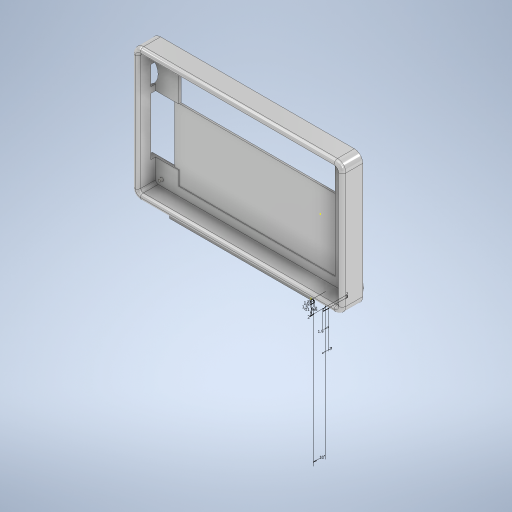
# Autodesk Inventor part: monitor-stand
Saved by Autodesk Inventor 2023 (Build 270158030, 158C)
## iProperties
Created: 2024-02-27
Part Number: monitor-stand
Material: Generic
Document SubType Name: Modeling
Designer: Imogen Heard
Density: 1 g/cm^3
Appearance: Expanded Metal 01
Author: Imogen Heard
Autodesk Inventor part; units mm, degrees
ref_plane "YZ Plane" through (0, 0, 0) normal (1, 0, 0) x (0, 1, 0)
ref_plane "XZ Plane" through (0, 0, 0) normal (0, 1, 0) x (-1, 0, 0)
ref_plane "XY Plane" through (0, 0, 0) normal (0, 0, 1) x (1, 0, 0)
sketch "Sketch1" plane through (0, 0, 0) normal (0, 0, 1) x (1, 0, 0)
  line L0 (-82.5, 50) -> (82.5, 50)
  line L1 (82.5, 50) -> (82.5, -50)
  line L2 (82.5, -50) -> (-82.5, -50)
  line L3 (-82.5, -50) -> (-82.5, 50)
  point P0 (0, 0)
  dimension "d0" = 165
  dimension "d1" = 100
  dimension "d2" = 82.5
  dimension "d3" = 50
  constraints: 8 end point, 2 parallel, 1 horizontal, 1 perpendicular
  measures "d0" distance between parallel lines of L1 L3
  measures "d1" distance between parallel lines of L2 L0
  measures "d2" horizontal distance of L2.end point (0, 0)
  measures "d3" distance from line of L2 point (0, 0)
extrude "Extrusion1" add sketch "Sketch1" along normal blind 8.36
sketch "Sketch2" plane through (0, 0, 0) normal (0, 0, -1) x (-1, 0, 0)
  circle A0 centre (-77.5, 45) radius 2.75
  circle A1 centre (77.5, 45) radius 2.75
  circle A2 centre (77.5, -45) radius 2.75
  circle A3 centre (-77.5, -45) radius 2.75
  line L0 (-82.5, 50) -> (82.5, 50) projected
  line L1 (-82.5, -50) -> (-82.5, 50) projected
  line L2 (82.5, -50) -> (-82.5, -50) projected
  line L3 (82.5, 50) -> (82.5, -50) projected
  point P0 (0, 0)
  dimension "d6" = 5.5
  dimension "d7" = 5
  dimension "d8" = 5
  dimension "d9" = 5
  dimension "d10" = 5
  constraints: 4 centre point, 3 equal radius, 2 horizontal alignment, 2 vertical alignment
  measures "d6" diameter of A3
  measures "d7" distance from line of L0 A0.centre
  measures "d8" distance from line of L1 A0.centre
  measures "d9" distance from line of L2 A3.centre
  measures "d10" distance from line of L3 A2.centre
extrude "Extrusion2" add sketch "Sketch2" along normal blind 4 contours A0 | A1 | A2 | A3
hole "Hole1" at (-77.5, -45, -4) direction (0, 0, 1) diameter 2.013 depth 4 tip angle 118 start extended yes countersink diameter 4 countersink angle 90 thread size "M2.5x0.45" class "6H" standard "ISO Metric profile"
hole "Hole2" at (77.5, 45, -4) direction (0, 0, 1) diameter 2.013 depth 4 tip angle 118 start extended yes countersink diameter 4 countersink angle 90 thread size "M2.5x0.45" class "6H" standard "ISO Metric profile"
hole "Hole3" at (77.5, -45, -4) direction (0, 0, 1) diameter 2.013 depth 4 tip angle 118 start extended yes countersink diameter 4 countersink angle 90 thread size "M2.5x0.45" class "6H" standard "ISO Metric profile"
hole "Hole4" at (-77.5, 45, -4) direction (0, 0, 1) diameter 2.013 depth 4 tip angle 118 start extended yes countersink diameter 4 countersink angle 90 thread size "M2.5x0.45" class "6H" standard "ISO Metric profile"
fillet "Fillet1" radius 2 4 edges at (82.5, 50, 4.18) (-82.5, 50, 4.18) (82.5, -50, 4.18) (-82.5, -50, 4.18)
sketch "Sketch4" plane through (0, 0, 0) normal (0, 0, -1) x (-1, 0, 0)
  line L0 (81.5, 35) -> (73.35, 35)
  line L1 (73.35, 35) -> (73.35, 23)
  line L2 (73.35, 23) -> (81.5, 23)
  line L3 (81.5, 23) -> (81.5, 35)
  line L4 (-80.5, 50) -> (80.5, 50) projected
  line L5 (82.5, 48) -> (82.5, -48) projected
  point P0 (0, 0)
  dimension "d54" = 15
  dimension "d55" = 12
  dimension "d56" = 9.15
  dimension "d57" = 1
  constraints: 8 end point, 2 parallel, 1 horizontal, 1 perpendicular
  measures "d54" distance between parallel lines of L0 L4
  measures "d55" distance between parallel lines of L2 L0
  measures "d56" distance between parallel lines of L5 L1
  measures "d57" distance between parallel lines of L5 L3
extrude "Extrusion3" add sketch "Sketch4" along normal blind 3
fillet "Fillet2" radius 6 2 edges at (-81.5, 35, -1.5) (-81.5, 23, -1.5)
sketch "Sketch5" plane through (0, 0, 0) normal (0, 0, -1) x (-1, 0, 0)
  arc A0 (77.425, 21.5) -> (77.425, 36.5) centre (77.425, 29) ccw
  line L0 (73.35, 35) -> (73.35, 23) projected
  line L1 (73.35, 23) -> (75.5, 23) projected
  line L2 (75.5, 35) -> (73.35, 35) projected
  line L3 (81.5, 35) -> (73.35, 35) projected
  line L4 (77.425, 36.5) -> (77.425, 21.5)
  arc A1 (75.5, 23) -> (75.5, 35) centre (75.5, 29) ccw projected
  point P0 (0, 0)
  point P1 (77.425, 35)
  point P2 (77.425, 35)
  point P3 (77.425, 23)
  point P4 (77.425, 34.6828)
  point P5 (77.425, 23.3172)
  point P6 (77.425, 35)
  dimension "d60" = 15
  dimension "d61" = 12
  dimension "d62" = 6
  dimension "d64" = 4.075
  constraints: 2 end point, 2 point on circle, 1 centre point, 1 midpoint
  measures "d60" diameter of A0
  measures "d61" distance from line of point (77.425, 35) L1
  measures "d62" distance from line of L1 A0.centre
  measures "d64" distance from line of L0 A0.centre
extrude "Extrusion4" add sketch "Sketch5" along normal blind 2.7 contours L4 A1 A0 | L4 A1
sketch "Sketch6" plane through (-82.5, -48, 8.36) normal (-1, 0, 0) x (0, 0, 1)
  line L0 (-14.66, 18.5) -> (-10.47, 18.5)
  line L1 (-10.47, 33.5) -> (-14.66, 33.5)
  line L2 (-14.66, 33.5) -> (-14.66, 18.5)
  line L3 (-10.47, 20) -> (-9.06, 21)
  line L4 (-9.06, 21) -> (-9.06, 31)
  line L5 (-8.36, 0) -> (-8.36, 96) projected
  line L6 (-9.06, 31) -> (-10.47, 32)
  line L7 (-10.47, 33) -> (-8.36, 33)
  line L8 (-8.36, 33) -> (-8.36, 33.5)
  line L9 (-8.36, 33.5) -> (-10.47, 33.5)
  line L10 (-10.47, 18.5) -> (-8.36, 18.5)
  line L11 (-8.36, 18.5) -> (-8.36, 19)
  line L12 (-8.36, 19) -> (-10.47, 19)
  line L13 (-8.36, -2) -> (0, -2) projected
  line L14 (-10.47, 19) -> (-10.47, 20)
  line L15 (-10.47, 32) -> (-10.47, 33)
  line L16 (-10.92, 33.05) -> (-10.92, 31.7675)
  line L17 (-10.92, 31.7675) -> (-9.51, 30.7675)
  line L18 (-9.51, 30.7675) -> (-9.51, 21.2325)
  line L19 (-9.51, 21.2325) -> (-10.92, 20.2325)
  line L20 (-10.92, 20.2325) -> (-10.92, 18.95)
  line L21 (-10.92, 18.95) -> (-14.21, 18.95)
  line L22 (-14.21, 18.95) -> (-14.21, 33.05)
  line L23 (-14.21, 33.05) -> (-10.92, 33.05)
  point P0 (-8.36, 48)
  point P1 (-12.565, 33.05)
  point P2 (-10.47, 32.5)
  point P3 (-10.47, 19.5)
  point P4 (-8.36, 18.5)
  point P5 (-10.47, 33.5)
  dimension "d68" = 0.5
  dimension "d69" = 0.5
  dimension "d70" = 15
  dimension "d71" = 6.3
  dimension "d73" = 0.7
  dimension "d74" = 1.5
  dimension "d75" = 1.5
  dimension "d76" = 20.5
  dimension "d77" = 2.5
  dimension "d78" = 2.5
  dimension "d79" = 2.11
  dimension "d80" = 0.45
  dimension "d81" = 0.45
  dimension "d82" = 0.45
  dimension "d83" = 0.45
  dimension "d84" = 0.45
  dimension "d85" = 0.45
  constraints: 44 end point, 9 parallel, 6 perpendicular, 3 horizontal, 3 midpoint, 2 point on line, 1 coincident, 1 vertical alignment, 2 other
  measures "d68" distance between parallel lines of L9 L7
  measures "d69" distance between parallel lines of L12 L10
  measures "d70" distance between parallel lines of L1 L0
  measures "d71" distance between parallel lines of L5 L2
  measures "d73" distance between parallel lines of L5 L4
  measures "d74" distance from line of L1 L6.end
  measures "d75" distance from line of L0 L3.start
  measures "d76" distance between parallel lines of L13 L0
  measures "d77" distance from line of L1 L4.end
  measures "d78" distance from line of L0 L3.end
  measures "d79" distance between parallel lines of L5 L15
  measures "d80" distance between parallel lines of L2 L22
  measures "d81" distance from line of L1 point (-12.565, 33.05)
  measures "d82" distance between parallel lines of L4 L18
  measures "d83" distance from line of point (-10.47, 32.5) L16
  measures "d84" distance between parallel lines of L0 L21
  measures "d85" distance from line of point (-10.47, 19.5) L20
extrude "Extrusion5" add sketch "Sketch6" along normal blind 0.4 and the other way blind 12 contours L2 L1 L9 L5 L7 L15 L6 L4 L3 L14 L12 L10 L0
fillet "Fillet3" radius 0.5 6 edges at (-76.7, -14.5, -6.3) (-76.7, -29.5, -6.3) (-76.7, -27.7675, -2.56) (-76.7, -16.2325, -2.56) (-76.7, -17, -0.7) (-76.7, -27, -0.7)
fillet "Fillet4" radius 0.2 8 edges at (-76.7, -29.05, -5.85) (-76.7, -14.95, -5.85) (-76.7, -29.05, -2.56) (-76.7, -26.7675, -1.15) (-76.7, -17.2325, -1.15) (-76.7, -14.95, -2.56) (-76.7, -16, -2.11) (-76.7, -28, -2.11)
sketch "Sketch7" plane through (-70.5, -48, 8.36) normal (-1, 0, 0) x (0, 0, -1)
  arc A0 (9.2708, -20.8505) -> (9.06, -21.2584) centre (9.56, -21.2584) ccw projected
  line L0 (10.3857, -20.0598) -> (9.2708, -20.8505) projected
  arc A1 (10.3857, -20.0598) -> (10.47, -19.8967) centre (10.27, -19.8967) ccw projected
  line L1 (10.47, -19) -> (10.47, -19.8967) projected
  line L2 (8.36, -19) -> (10.47, -19) projected
  line L3 (14.16, -18.5) -> (8.36, -18.5) projected
  arc A2 (14.66, -19) -> (14.16, -18.5) centre (14.16, -19) ccw projected
  line L4 (14.66, -33) -> (14.66, -19) projected
  arc A3 (14.16, -33.5) -> (14.66, -33) centre (14.16, -33) ccw projected
  line L5 (8.36, -33.5) -> (14.16, -33.5) projected
  line L6 (10.47, -33) -> (8.36, -33) projected
  line L7 (10.47, -32.1033) -> (10.47, -33) projected
  arc A4 (10.47, -32.1033) -> (10.3857, -31.9402) centre (10.27, -32.1033) ccw projected
  line L8 (9.2708, -31.1495) -> (10.3857, -31.9402) projected
  arc A5 (9.06, -30.7416) -> (9.2708, -31.1495) centre (9.56, -30.7416) ccw projected
  line L9 (9.06, -21.2584) -> (9.06, -30.7416) projected
  arc A6 (10.92, -32.0258) -> (10.7092, -31.618) centre (10.42, -32.0258) ccw projected
  line L10 (10.92, -32.85) -> (10.92, -32.0258) projected
  arc A7 (10.92, -32.85) -> (11.12, -33.05) centre (11.12, -32.85) ccw projected
  line L11 (14.01, -33.05) -> (11.12, -33.05) projected
  arc A8 (14.01, -33.05) -> (14.21, -32.85) centre (14.01, -32.85) ccw projected
  line L12 (14.21, -19.15) -> (14.21, -32.85) projected
  arc A9 (14.21, -19.15) -> (14.01, -18.95) centre (14.01, -19.15) ccw projected
  line L13 (11.12, -18.95) -> (14.01, -18.95) projected
  arc A10 (11.12, -18.95) -> (10.92, -19.15) centre (11.12, -19.15) ccw projected
  line L14 (10.92, -19.9742) -> (10.92, -19.15) projected
  arc A11 (10.7092, -20.382) -> (10.92, -19.9742) centre (10.42, -19.9742) ccw projected
  line L15 (9.5943, -21.1727) -> (10.7092, -20.382) projected
  arc A12 (9.5943, -21.1727) -> (9.51, -21.3359) centre (9.71, -21.3359) ccw projected
  line L16 (9.51, -30.6641) -> (9.51, -21.3359) projected
  arc A13 (9.51, -30.6641) -> (9.5943, -30.8273) centre (9.71, -30.6641) ccw projected
  line L17 (10.7092, -31.618) -> (9.5943, -30.8273) projected
  line L18 (8.36, -33) -> (8.36, -33.5) projected
  line L19 (8.36, -18.5) -> (8.36, -19) projected
  point P0 (8.36, -48)
extrude "Extrusion6" add sketch "Sketch7" along normal blind 4.5 contours A6 L17 A13 L16 A12 L15 A11 L14 A10 L13 A9 L12 A8 L11 A7 L10
sketch "Sketch8" plane through (-82.5, -48, 8.36) normal (-1, 0, 0) x (0, 0, 1)
  line L0 (-10.06, 42.6) -> (-10.06, 48.5) construction
  line L1 (-8.46, 42.6) -> (-8.46, 48.5)
  line L2 (-11.66, 48.5) -> (-11.66, 42.6)
  arc A0 (-11.66, 42.6) -> (-8.46, 42.6) centre (-10.06, 42.6) ccw
  arc A1 (-8.46, 48.5) -> (-11.66, 48.5) centre (-10.06, 48.5) ccw
  line L3 (-8.36, 71.4778) -> (-8.36, 33.5) projected
  line L4 (-11.31, 42.6) -> (-11.31, 48.5)
  arc A2 (-8.81, 48.5) -> (-11.31, 48.5) centre (-10.06, 48.5) ccw
  line L5 (-8.81, 48.5) -> (-8.81, 42.6)
  arc A3 (-11.31, 42.6) -> (-8.81, 42.6) centre (-10.06, 42.6) ccw
  point P0 (-8.36, 48)
  point P1 (-10.06, 45.55)
  point P2 (-10.06, 50.1)
  point P3 (-10.06, 41)
  point P4 (-8.36, -2)
  dimension "d94" = 9.1
  dimension "d95" = 3.2
  dimension "d96" = 0.1
  dimension "d97" = 43
  dimension "d98" = 0.35
  constraints: 12 end point, 10 point on circle, 4 centre point, 4 tangent, 2 parallel, 1 midpoint, 1 vertical, 3 other
  measures "d94" distance of point (-10.06, 50.1) point (-10.06, 41)
  measures "d95" distance between parallel lines of L1 L2
  measures "d96" distance between parallel lines of L3 L1
  measures "d97" vertical distance of point (-8.36, -2) point (-10.06, 41)
  measures "d98" distance between parallel lines of L2 L4
extrude "Extrusion7" add sketch "Sketch8" against normal blind 7.5
sketch "Sketch9" plane through (-75, -48, 8.36) normal (1, 0, 0) x (0, 0, -1)
  arc A0 (11.66, 48.5) -> (8.46, 48.5) centre (10.06, 48.5) ccw projected
  line L0 (8.46, 48.5) -> (8.46, 42.6) projected
  arc A1 (8.46, 42.6) -> (11.66, 42.6) centre (10.06, 42.6) ccw projected
  line L1 (11.66, 42.6) -> (11.66, 48.5) projected
  line L2 (8.81, 42.6) -> (8.81, 48.5) projected
  arc A2 (11.31, 48.5) -> (8.81, 48.5) centre (10.06, 48.5) ccw projected
  line L3 (11.31, 48.5) -> (11.31, 42.6) projected
  arc A3 (8.81, 42.6) -> (11.31, 42.6) centre (10.06, 42.6) ccw projected
  point P0 (8.36, 48)
extrude "Extrusion8" add sketch "Sketch9" against normal blind 2 contours L2 A2 L3 A3
sketch "Sketch10" plane through (-82.5, -48, 8.36) normal (-1, 0, 0) x (0, 0, 1)
  circle A0 centre (-10.91, 59) radius 2.45
  circle A1 centre (-10.91, 59) radius 1.72
  line L0 (-8.36, 71.4778) -> (-8.36, 33.5) projected
  line L1 (0, 98) -> (-8.36, 98) projected
  point P0 (-8.36, 48)
  dimension "d103" = 4.9
  dimension "d104" = 0.73
  dimension "d105" = 2.55
  dimension "d106" = 39
  constraints: 2 centre point, 1 concentric
  measures "d103" diameter of A0
  measures "d104" radial gap between concentric circles of A0 A1
  measures "d105" distance from line of L0 A0.centre
  measures "d106" distance from line of L1 A0.centre
extrude "Extrusion9" add sketch "Sketch10" against normal blind 14
sketch "Sketch11" plane through (-68.5, 11, -2.55) normal (1, 0, 0) x (0, 0, -1)
  line L0 (-2.55, 12.4778) -> (-2.55, -25.5) projected
  line L1 (2.45, 3.175) -> (-2.55, 3.175)
  line L2 (-2.55, 3.175) -> (-2.55, -3.175)
  line L3 (-2.55, -3.175) -> (2.45, -3.175)
  line L4 (2.45, -3.175) -> (2.45, 3.175)
  circle A0 centre (0, 0) radius 1.72 projected
  point P0 (-2.55, -11)
  point P1 (-2.55, 3.175)
  dimension "d109" = 6.35
  dimension "d110" = 3.175
  dimension "d111" = 5
  constraints: 8 end point, 2 parallel, 1 horizontal, 1 perpendicular, 1 point on line
  measures "d109" distance between parallel lines of L3 L1
  measures "d110" distance from line of A0.centre L3
  measures "d111" distance between parallel lines of L0 L4
extrude "Extrusion10" add sketch "Sketch11" against normal blind 12
sketch "Sketch12" plane through (0, 0, 0) normal (0, 0, -1) x (-1, 0, 0)
  line L0 (-63.9, 42.33) -> (-25.9, 42.33)
  line L1 (-25.9, 42.33) -> (-25.9, 24.33)
  line L2 (-25.9, 24.33) -> (-63.9, 24.33)
  line L3 (-63.9, 24.33) -> (-63.9, 42.33)
  line L4 (22.83, 42.33) -> (60.83, 42.33)
  line L5 (60.83, 42.33) -> (60.83, 24.33)
  line L6 (60.83, 24.33) -> (22.83, 24.33)
  line L7 (22.83, 24.33) -> (22.83, 42.33)
  line L8 (-82.5, -48) -> (-82.5, 48) projected
  line L9 (-80.5, 50) -> (80.5, 50) projected
  line L10 (82.5, 48) -> (82.5, 34.5222) projected
  point P0 (0, 0)
  dimension "d114" = 38
  dimension "d115" = 18
  dimension "d116" = 38
  dimension "d117" = 18.6
  dimension "d118" = 7.67
  dimension "d119" = 21.67
  constraints: 16 end point, 4 parallel, 2 horizontal, 2 horizontal alignment, 2 perpendicular, 2 point on line
  measures "d114" distance between parallel lines of L1 L3
  measures "d115" distance between parallel lines of L2 L0
  measures "d116" distance between parallel lines of L5 L7
  measures "d117" distance between parallel lines of L8 L3
  measures "d118" distance between parallel lines of L9 L0
  measures "d119" distance between parallel lines of L5 L10
extrude "Extrusion11" add sketch "Sketch12" along normal blind 5.09
fillet "Fillet5" radius 3 8 edges at (63.9, 24.33, -2.545) (63.9, 42.33, -2.545) (25.9, 24.33, -2.545) (25.9, 42.33, -2.545) (-60.83, 42.33, -2.545) (-22.83, 42.33, -2.545) (-22.83, 24.33, -2.545) (-60.83, 24.33, -2.545)
fillet "Fillet6" radius 0.2 16 edges at (-23.7087, 41.4513, -5.09) (-22.83, 33.33, -5.09) (-23.7087, 25.2087, -5.09) (-41.83, 24.33, -5.09) (-59.9513, 25.2087, -5.09) (-60.83, 33.33, -5.09) (-59.9513, 41.4513, -5.09) (-41.83, 42.33, -5.09) (26.7787, 41.4513, -5.09) (44.9, 42.33, -5.09) (63.0213, 41.4513, -5.09) (63.9, 33.33, -5.09) (63.0213, 25.2087, -5.09) (44.9, 24.33, -5.09) (26.7787, 25.2087, -5.09) (25.9, 33.33, -5.09)
sketch "Sketch13" plane through (77.5, 45, -4) normal (0, 0, -1) x (-1, 0, 0)
  line L0 (-10, 10) -> (165, 10)
  line L1 (165, 10) -> (165, -100)
  line L2 (165, -100) -> (-10, -100)
  line L3 (-10, -100) -> (-10, 10)
  line L4 (-3, 5) -> (158, 5) projected
  line L5 (-5, -93) -> (-5, 3) projected
  line L6 (160, -21.5222) -> (160, -59.5) projected
  line L7 (158, -95) -> (-3, -95) projected
  line L8 (11, -2) -> (141, -2)
  line L9 (141, -88) -> (11, -88)
  line L10 (141, -88) -> (141, -2)
  line L11 (141, -29.8869) -> (141, -2)
  line L12 (160, 3) -> (160, -93) projected
  line L13 (160, -39.175) -> (160, -57.5)
  line L14 (160, -74.5) -> (160, -93) projected
  line L15 (11, -2) -> (11, -88)
  line L16 (146, -37.175) -> (146, -30.825) projected
  line L17 (144, -28.825) -> (144, -39.175)
  line L18 (146, -57.5) -> (146, -76.5)
  line L19 (146, -30.825) -> (158, -30.825) projected
  line L20 (146, -37.175) -> (158, -37.175) projected
  line L21 (160.4, -59.5) -> (148, -59.5) projected
  line L22 (148, -74) -> (148, -60) projected
  line L23 (160, -74.5) -> (148, -74.5) projected
  line L24 (144, -28.825) -> (165, -28.825)
  line L25 (144, -39.175) -> (165, -39.175)
  line L26 (146, -76.5) -> (165, -76.5)
  line L27 (146, -57.5) -> (165, -57.5)
  arc A0 (165, -6) -> (165, -26) centre (169.6, -16) ccw
  line L28 (150.85, -10) -> (150.85, -22) projected
  line L29 (141, -28.825) -> (160, -28.825)
  line L30 (160, -28.825) -> (160, -76.5)
  line L31 (160, -76.5) -> (141, -76.5)
  line L32 (141, -76.5) -> (141, -28.825)
  point P0 (77.5, -45)
  point P1 (-10, -45)
  point P2 (154.5, -39.175)
  point P3 (160, -57.5)
  point P4 (160, -39.175)
  point P5 (160, -28.825)
  point P6 (150.85, -16)
  dimension "d124" = 5
  dimension "d125" = 5
  dimension "d126" = 5
  dimension "d127" = 5
  dimension "d128" = 12
  dimension "d130" = 12
  dimension "d134" = 16
  dimension "d135" = 19
  dimension "d139" = 2
  dimension "d141" = 2
  dimension "d143" = 2
  dimension "d145" = 2
  dimension "d146" = 2
  dimension "d147" = 2
  dimension "d175" = 16
  dimension "d176" = 10
  dimension "d177" = 10
  dimension "d178" = 4.6
  constraints: 40 end point, 8 parallel, 8 point on line, 5 perpendicular, 3 horizontal, 3 midpoint, 2 horizontal alignment, 2 point on circle, 2 vertical alignment, 1 centre point
  measures "d124" distance between parallel lines of L0 L4
  measures "d125" distance between parallel lines of L3 L5
  measures "d126" distance between parallel lines of L1 L6
  measures "d127" distance between parallel lines of L7 L2
  measures "d128" distance between parallel lines of L8 L0
  measures "d130" distance between parallel lines of L2 L9
  measures "d134" distance between parallel lines of L5 L15
  measures "d135" distance between parallel lines of L12 L11
  measures "d139" distance between parallel lines of L17 L16
  measures "d141" distance between parallel lines of L18 L22
  measures "d143" distance between parallel lines of L24 L19
  measures "d145" distance from line of point (154.5, -39.175) L20
  measures "d146" distance between parallel lines of L27 L21
  measures "d147" distance between parallel lines of L26 L23
  measures "d175" distance from line of L0 A0.start
  measures "d176" vertical distance of point (150.85, -16) A0.start
  measures "d177" vertical distance of A0.end point (150.85, -16)
  measures "d178" horizontal distance of A0.start A0.centre
extrude "Extrusion12" add sketch "Sketch13" along normal blind 2 separate body contours L0 L1 A0 L12 L6 L24 L29 L10 L8 L15 L9 L31 L26 L2 L3 | L1 L24 L6 L12 A0
sketch "Sketch14" plane through (77.5, 45, -4) normal (0, 0, 1) x (1, 0, 0)
  line L0 (-165, -6) -> (-165, 10) projected
  line L1 (10, -100) -> (-165, -100) projected
  line L2 (10, 10) -> (10, -100) projected
  line L3 (-165, 10) -> (10, 10) projected
  line L4 (-11, -2) -> (-141, -2) projected
  line L5 (-11, -88) -> (-11, -2) projected
  line L6 (-141, -88) -> (-11, -88) projected
  line L7 (-141, -2) -> (-141, -28.825) projected
  arc A0 (-160, -93) -> (-158, -95) centre (-158, -93) ccw projected
  line L8 (-158, -95) -> (3, -95) projected
  arc A1 (3, -95) -> (5, -93) centre (3, -93) ccw projected
  line L9 (5, -93) -> (5, 3) projected
  arc A2 (5, 3) -> (3, 5) centre (3, 3) ccw projected
  line L10 (3, 5) -> (-158, 5) projected
  arc A3 (-158, 5) -> (-160, 3) centre (-158, 3) ccw projected
  line L11 (-160, 3) -> (-160, -93) projected
  arc A4 (-160, -10.4778) -> (-160, -21.5222) centre (-154.925, -16) ccw projected
  line L12 (-160, -10.4778) -> (-160, -21.5222) projected
  arc A5 (-160, -10.4778) -> (-160, -21.5222) centre (-154.925, -16) ccw projected
  line L13 (-160.4, -71.7416) -> (-160.4, -62.2584) projected
  line L14 (-141, -2) -> (-141, -88) projected
  circle A6 centre (-155, 0) radius 2.75 projected
  line L15 (-158, 5.2) -> (3, 5.2)
  arc A7 (5.2, 3) -> (3, 5.2) centre (3, 3) ccw
  line L16 (5.2, 3) -> (5.2, -93)
  arc A8 (3, -95.2) -> (5.2, -93) centre (3, -93) ccw
  line L17 (3, -95.2) -> (-158, -95.2)
  arc A9 (-160.2, -93) -> (-158, -95.2) centre (-158, -93) ccw
  arc A10 (-158, 5.2) -> (-160.2, 3) centre (-158, 3) ccw
  line L18 (-160.2, -24) -> (-165, -24)
  line L19 (-165, -8) -> (-160.2, -8)
  line L20 (-160.2, -10.6685) -> (-160.2, -21.3315)
  line L21 (-160.2, -8) -> (-160.2, 3)
  line L22 (-160.2, -21.3315) -> (-160.2, -10.6685)
  line L23 (-160.2, -28.825) -> (-160.2, -24)
  line L24 (-160.2, -93) -> (-160.2, -76.5)
  line L25 (-160.2, -57.5) -> (-160.2, -39.175)
  arc A11 (-165, -26) -> (-165, -6) centre (-169.6, -16) ccw projected
  line L26 (-165, -28.825) -> (-165, -26) projected
  line L27 (-141, -28.825) -> (-165, -28.825) projected
  line L28 (-165, -76.5) -> (-141, -76.5) projected
  line L29 (-165, -100) -> (-165, -76.5) projected
  line L30 (-141, -76.5) -> (-141, -88) projected
  point P0 (-77.5, -45)
  point P1 (-162.425, -16)
  point P2 (-162.425, -16)
  point P3 (-165, -8)
  point P4 (-162.0396, -24)
  point P5 (-162.0396, -8)
  dimension "d148" = 0.2
  dimension "d149" = 8
  dimension "d150" = 8
  dimension "d151" = 0.2
  dimension "d152" = 0.2
  dimension "d153" = 0.2
  constraints: 22 end point, 12 point on circle, 4 centre point, 4 vertical alignment, 1 horizontal, 1 parallel, 5 other
  measures "d148" distance between parallel lines of L10 L15
  measures "d149" distance from line of point (-162.425, -16) L18
  measures "d150" distance from line of L19 point (-162.425, -16)
  measures "d151" distance between parallel lines of L11 L23
  measures "d152" distance between parallel lines of L11 L21
  measures "d153" radial gap between concentric circles of A3 A10
extrude "Extrusion13" add sketch "Sketch14" along normal blind 15 contours L0 L3 L2 L1 L29 L28 L24 A9 L17 A8 L16 A7 L15 A10 L21 L19 A11 | L18 L23 L27 L26 A11 bodies 2
sketch "Sketch15" plane through (77.5, 45, -6) normal (0, 0, -1) x (-1, 0, 0)
  circle A0 centre (155, -90) radius 2 projected
  circle A1 centre (155, 0) radius 2.75 projected
  circle A2 centre (0, -90) radius 2.75 projected
  circle A3 centre (0, 0) radius 2.75 projected
  point P0 (77.5, -45)
hole "Hole6" at (77.5, 45, -6) at (77.5, -45, -6) at (-77.5, -45, -6) at (-77.5, 45, -6) direction (0, 0, 1) diameter 2.9 depth 8.1 tip angle 118 start extended yes counterbore diameter 5.5 counterbore depth 0.5 bodies 2 clearance for "Countersunk Raised Head Screw ISO 2010" size "M2.5" standard "DIN"
fillet "Fillet7" radius 7 4 edges at (-87.5, 55, 2.5) (-87.5, -55, 2.5) (87.5, -55, 2.5) (87.5, 55, 2.5)
sketch "Sketch16" plane through (-87.5, -31.5, -6) normal (0, 1, 0) x (1, 0, 0)
  line L0 (4.8, -2) -> (24, -2) projected
  line L1 (0, 0) -> (24, 0) projected
  line L2 (0, -17) -> (0, 0) projected
  line L3 (4.8, -17) -> (0, -17) projected
  line L4 (4.8, -2) -> (4.8, -17) projected
  line L5 (4.8, -2) -> (4.8, -17) projected
  line L6 (0, -17) -> (0, 0) projected
  line L7 (4.8, -17) -> (0, -17)
  line L8 (0, -17) -> (0, -6)
  line L9 (0, -6) -> (4.8, -6)
  line L10 (4.8, -6) -> (4.8, -17)
  line L11 (24, -2) -> (24, 0) projected
  point P0 (87.5, -6)
  point P1 (4.6, -6)
  constraints: 8 end point, 2 parallel, 1 horizontal, 1 horizontal alignment, 1 perpendicular, 1 point on line
extrude "Extrusion14" add sketch "Sketch16" along normal blind 73 contours L4 L3 L2 L9 bodies 2
chamfer "Chamfer1" [suppressed]
fillet "Fillet8" radius 3 8 edges at (-85.4497, -52.9497, 11) (0, -55, 11) (85.4497, -52.9497, 11) (87.5, 0, 11) (85.4497, 52.9497, 11) (0, 55, 11) (-85.4497, 52.9497, 11) (-87.5, 0, 11)
fillet "Fillet9" radius 3 8 edges at (-82.0556, 49.5556, 11) (0, 50.2, 11) (82.0556, 49.5556, 11) (82.7, 0, 11) (82.0556, -49.5556, 11) (0, -50.2, 11) (-82.0556, -49.5556, 11) (-82.7, 0, 11)
sketch "Sketch17" plane through (-77.5, 45, -4) normal (0, 0, -1) x (-1, 0, 0)
  circle A0 centre (0, 0) radius 1.0065 projected
  circle A1 centre (-155, 0) radius 1.0065 projected
  circle A2 centre (-155, -90) radius 1.0065 projected
  circle A3 centre (0, -90) radius 1.0065 projected
  point P0 (-77.5, -45)
extrude "Extrusion15" add sketch "Sketch17" along normal blind 7.3 and the other way blind 2 separate body
sketch "Sketch18" plane through (-77.5, 45, -11.3) normal (0, 0, -1) x (-1, 0, 0)
  circle A0 centre (0, 0) radius 2.08
  circle A1 centre (0, 0) radius 1.0065 projected
  circle A2 centre (0, -90) radius 2.08
  circle A3 centre (-155, -90) radius 2.08
  circle A4 centre (-155, 0) radius 2.08
  circle A5 centre (-155, 0) radius 1.0065 projected
  circle A6 centre (-155, -90) radius 1.0065 projected
  circle A7 centre (0, -90) radius 1.0065 projected
  point P0 (-77.5, -45)
  dimension "d190" = 4.16
  constraints: 4 centre point, 4 concentric, 3 equal radius
  measures "d190" diameter of A0
extrude "Extrusion16" add sketch "Sketch18" along normal blind 1.4 contours A0 | A1 | A2 | A3 | A4 | A5 | A6 | A7 bodies 3
fillet "Fillet10" radius 0.6 8 edges at (79.58, -45, -12.7) (79.58, -45, -11.3) (-75.42, -45, -12.7) (-75.42, -45, -11.3) (79.58, 45, -11.3) (79.58, 45, -12.7) (-75.42, 45, -12.7) (-75.42, 45, -11.3)
fillet "Fillet11" radius 4 1 edges at (-81.0927, 29, -6)
sketch "Sketch19" plane through (77.5, 45, -6) normal (0, 0, -1) x (-1, 0, 0)
  line L0 (11, -88) -> (11, -2) projected
  line L1 (141, -2) -> (141, -28.825) projected
  line L2 (11, -88) -> (141, -88)
  line L3 (141, -88) -> (141, -28.825)
  line L4 (141, -28.825) -> (11, -28.825)
  line L5 (11, -28.825) -> (11, -88)
  line L6 (160.2, -76.5) -> (141, -76.5) projected
  line L7 (141, -28.825) -> (145, -28.825)
  line L8 (145, -28.825) -> (145, -76.5)
  line L9 (145, -76.5) -> (141, -76.5)
  line L10 (141, -76.5) -> (141, -28.825)
  point P0 (77.5, -45)
  dimension "d197" = 4
  constraints: 16 end point, 4 parallel, 2 horizontal, 2 perpendicular, 1 point on line
  measures "d197" distance between parallel lines of L8 L3
extrude "Extrusion17" add sketch "Sketch19" against normal blind 1.4 bodies 2
sketch "Sketch20" plane through (77.5, 45, -6) normal (0, 0, -1) x (-1, 0, 0)
  line L0 (-5, -82.55) -> (160, -82.55)
  line L1 (160, -82.55) -> (160, -103)
  line L2 (160, -103) -> (-5, -103)
  line L3 (-5, -103) -> (-5, -82.55)
  circle A0 centre (0, -90) radius 1.45 projected
  circle A1 centre (155, -90) radius 1.45 projected
  line L4 (-3, -100) -> (158, -100) projected
  point P0 (77.5, -45)
  dimension "d198" = 5
  dimension "d199" = 5
  dimension "d200" = 6
  dimension "d201" = 3
  constraints: 8 end point, 2 parallel, 1 horizontal, 1 perpendicular
  measures "d198" distance from line of L3 A0.centre
  measures "d199" distance from line of A1.centre L1
  measures "d200" distance edge to line of A1 L0
  measures "d201" distance between parallel lines of L2 L4
extrude "Extrusion18" add sketch "Sketch20" along normal blind 3 separate body
sketch "Sketch22" plane through (77.5, 45, -9) normal (0, 0, -1) x (-1, 0, 0)
  line L0 (160, -82.55) -> (-5, -82.55) projected
  line L1 (-5, -103) -> (160, -103) projected
  line L2 (10, -82.55) -> (-5, -82.55)
  line L3 (-5, -82.55) -> (-5, -103)
  line L4 (-5, -103) -> (10, -103)
  line L5 (10, -103) -> (10, -82.55)
  line L6 (160, -82.55) -> (145, -82.55)
  line L7 (145, -82.55) -> (145, -103)
  line L8 (145, -103) -> (160, -103)
  line L9 (160, -103) -> (160, -82.55)
  line L10 (141, -88) -> (11, -88) projected
  line L11 (-5, -103) -> (160, -103) projected
  line L12 (160, -103) -> (160, -82.55) projected
  line L13 (160, -82.55) -> (-5, -82.55) projected
  line L14 (-5, -82.55) -> (-5, -103) projected
  circle A0 centre (155, -90) radius 1.45 projected
  circle A1 centre (0, -90) radius 1.45 projected
  point P0 (77.5, -45)
  point P1 (10, -103)
  dimension "d204" = 15
  dimension "d205" = 15
  constraints: 16 end point, 4 parallel, 2 coincident, 2 horizontal, 2 perpendicular, 2 point on line
  measures "d204" distance between parallel lines of L9 L7
  measures "d205" distance between parallel lines of L3 L5
extrude "Extrusion19" add sketch "Sketch22" along normal blind 4.5 contours L9 L1 L7 L0 | L5 L1 L3 L0 bodies 4
sketch "Sketch23" plane through (77.5, 45, -13.5) normal (0, 0, -1) x (-1, 0, 0)
  circle A0 centre (0, -90) radius 1.45 projected
  circle A1 centre (155, -90) radius 1.45 projected
  point P0 (77.5, -45)
  constraints: 2 coincident
hole "Hole7" at (-77.5, -45, -13.5) at (77.5, -45, -13.5) direction (0, 0, 1) diameter 2.9 depth 9.6 tip angle 118 start extended yes counterbore diameter 5.5 counterbore depth 2 bodies 4 clearance for "Socket Head Cap Screw ISO 4762" size "M2.5" standard "ISO"
fillet "Fillet12" radius 10 8 edges at (82.5, -58, -9.75) (-82.5, -58, -9.75) (-82.5, -37.55, -9.75) (-67.5, -47.775, -9) (67.5, -47.775, -9) (82.5, -37.55, -9.75) (67.5, -47.775, -13.5) (-67.5, -47.775, -13.5)
sketch "Sketch24" plane through (77.5, 45, -6) normal (0, 0, 1) x (1, 0, 0)
  line L0 (-136.6484, -103) -> (-142.968, -103) projected
  line L1 (3, -100) -> (-158, -100) projected
  line L2 (-136.6484, -103) -> (-19.1801, -103)
  line L3 (-19.1801, -103) -> (-19.1801, -100)
  line L4 (-19.1801, -100) -> (-136.6484, -100)
  line L5 (-136.6484, -100) -> (-136.6484, -103)
  arc A0 (-162, -93) -> (-158, -97) centre (-158, -93) ccw projected
  line L6 (5, -92.55) -> (5, -93) projected
  point P0 (-77.5, -45)
  point P1 (-160.8284, -95.8284)
  point P2 (-136.6484, -101.5)
  point P3 (5, -92.775)
  dimension "d216" = 24.1801
  dimension "d217" = 24.1801
  constraints: 8 end point, 2 midpoint, 2 parallel, 1 horizontal, 1 perpendicular, 1 point on circle, 1 point on line
  measures "d216" horizontal distance of point (-160.828, -95.828) point (-136.648, -101.5)
  measures "d217" distance from line of L3 point (5, -92.775)
extrude "Extrusion20" add sketch "Sketch24" along normal blind 14 bodies 4
fillet "Fillet13" radius 3 20 edges at (-82.5, -47.775, -13.5) (-79.5711, -55.0711, -13.5) (-72.1438, -58, -13.5) (-68.4335, -58, -12.9207) (-62.5025, -58, -9.5793) (0, -58, -9) (62.5025, -58, -9.5793) (68.4335, -58, -12.9207) (72.1438, -58, -13.5) (79.5711, -55.0711, -13.5) (82.5, -47.775, -13.5) (79.5711, -40.4789, -13.5) (72.1438, -37.55, -13.5) (68.4335, -37.55, -12.9207) (62.5025, -37.55, -9.5793) (0, -37.55, -9) (-62.5025, -37.55, -9.5793) (-68.4335, -37.55, -12.9207) (-72.1438, -37.55, -13.5) (-79.5711, -40.4789, -13.5)
sketch "Sketch25" plane through (58.3199, -58, 8) normal (1, 0, 0) x (0, 0, -1)
  line L0 (0, 3) -> (0, 0) projected
  line L1 (0, 0) -> (2, 0)
  line L2 (2, 0) -> (2, -1.65)
  line L3 (2.7, -3.15) -> (0, -3.15)
  line L4 (0, -3.15) -> (0, 0)
  line L5 (2, -1.65) -> (2.7, -1.65)
  line L6 (2.7, -1.65) -> (2.7, -3.15)
  line L7 (14, 0) -> (0, 0) projected
  line L8 (12, 0) -> (15, 0)
  line L9 (15, 0) -> (15, -13.165)
  line L10 (15, -13.165) -> (10.1, -13.165)
  line L11 (12, -11.165) -> (12, 0)
  line L12 (10.1, -11.165) -> (12, -11.165)
  line L13 (10.1, -13.165) -> (10.1, -11.165)
  point P0 (8, 58)
  point P1 (2.35, -1.65)
  dimension "d221" = 0.7
  dimension "d222" = 1.65
  dimension "d223" = 2
  dimension "d225" = 10
  dimension "d226" = 11.165
  dimension "d227" = 3
  dimension "d228" = 2
  dimension "d229" = 1.9
  dimension "d230" = 1.5
  constraints: 25 end point, 4 horizontal, 4 parallel, 3 perpendicular, 2 coincident, 1 midpoint, 1 point on line
  measures "d221" distance between parallel lines of L2 L6
  measures "d222" distance between parallel lines of L7 L5
  measures "d223" distance between parallel lines of L2 L4
  measures "d225" distance between parallel lines of L11 L2
  measures "d226" distance between parallel lines of L12 L7
  measures "d227" distance between parallel lines of L9 L11
  measures "d228" distance between parallel lines of L10 L12
  measures "d229" distance between parallel lines of L11 L13
  measures "d230" distance from line of L3 point (2.35, -1.65)
equation "\"d2\" = 0.5 * d0"
equation "\"d3\" = 0.5 * d1"
equation "\"d64\" = 0.5 * d63"
equation "\"d110\" = 0.5 * d109"
equation "\"d116\" = d114"
equation "\"d151\" = d148"
equation "\"d152\" = d148"
equation "\"d153\" = d148"
equation "\"d63\" = 8.15"
body "Solid1"
